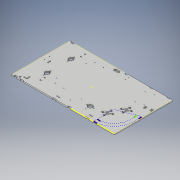
# Autodesk Inventor part: playfield
Saved by Autodesk Inventor 2017 (Build 210142000, 142)
## iProperties
Created: 2017-02-19
Part Number: playfield
Material: Generic
Document SubType Name: Modeling
Designer: John
Density: 1 g/cm^3
Appearance: Default
Author: John
Autodesk Inventor part; units mm, degrees
ref_plane "YZ Plane" through (0, 0, 0) normal (1, 0, 0) x (0, 1, 0)
ref_plane "XZ Plane" through (0, 0, 0) normal (0, 1, 0) x (-1, 0, 0)
ref_plane "XY Plane" through (0, 0, 0) normal (0, 0, 1) x (1, 0, 0)
sketch "Sketch2" plane through (0, 0, 0) normal (0, 1, 0) x (-1, 0, 0)
  line L0 (250, -141.5) -> (-250, -141.5)
  line L1 (-250, -141.5) -> (-250, 141.5)
  line L2 (-250, 141.5) -> (250, 141.5)
  line L3 (250, 141.5) -> (250, -141.5)
  line L4 (250, -141.5) -> (-250, 141.5) construction
  line L5 (-250, -141.5) -> (250, 141.5) construction
  line L6 (250, 138.5) -> (-250, 138.5) construction
  line L7 (250, 131.5) -> (-250, 131.5) construction
  line L8 (-250, 128.5) -> (250, 128.5) construction
  point P0 (0, 0)
  dimension "d0" = 500
  dimension "d1" = 283
  dimension "d4" = 3
  dimension "d5" = 7
  dimension "d6" = 3
  constraints: 18 end point, 6 point on line, 3 perpendicular, 2 horizontal, 2 midpoint, 2 parallel
  measures "d0" distance of L1.end L2.end
  measures "d1" distance of L0.end L1.end
  measures "d4" distance between parallel lines of L2 L6
  measures "d5" distance between parallel lines of L6 L7
  measures "d6" distance between parallel lines of L7 L8
extrude "Extrusion1" add sketch "Sketch2" along normal blind 6
sketch "Sketch3" plane through (0, 6, 0) normal (0, 1, 0) x (1, 0, 0)
  line L0 (-250, 141.5) -> (-250, -141.5) projected
  line L1 (-170, 66.5) -> (-170, -49.5) construction
  line L2 (-170, 66.5) -> (-170, 141.5) construction
  line L3 (250, 141.5) -> (-250, 141.5) construction
  line L4 (-170, -49.5) -> (-170, -141.5) construction
  line L5 (-250, -141.5) -> (250, -141.5) construction
  circle A0 centre (-170, 66.5) radius 10.825
  arc A1 (-169, 84.325) -> (-171, 84.325) centre (-170, 84.325) ccw
  line L6 (-170, 77.325) -> (-170, 84.325) construction
  line L7 (-169, 77.325) -> (-169, 84.325)
  line L8 (-171, 84.325) -> (-171, 77.325)
  arc A2 (-171, 77.325) -> (-169, 77.325) centre (-170, 77.325) ccw
  arc A3 (-169, 55.675) -> (-171, 55.675) centre (-170, 55.675) ccw
  line L9 (-169, 48.675) -> (-169, 55.675)
  arc A4 (-171, 48.675) -> (-169, 48.675) centre (-170, 48.675) ccw
  line L10 (-170, 55.675) -> (-170, 48.675) construction
  line L11 (-171, 55.675) -> (-171, 48.675)
  arc A5 (-169, -60.325) -> (-171, -60.325) centre (-170, -60.325) ccw
  arc A6 (-171, -38.675) -> (-169, -38.675) centre (-170, -38.675) ccw
  line L12 (-171, -31.675) -> (-171, -38.675)
  line L13 (-170, -38.675) -> (-170, -31.675) construction
  line L14 (-169, -38.675) -> (-169, -31.675)
  arc A7 (-169, -31.675) -> (-171, -31.675) centre (-170, -31.675) ccw
  circle A8 centre (-170, -49.5) radius 10.825
  arc A9 (-171, -67.325) -> (-169, -67.325) centre (-170, -67.325) ccw
  line L15 (-171, -60.325) -> (-171, -67.325)
  line L16 (-170, -60.325) -> (-170, -67.325) construction
  line L17 (-169, -67.325) -> (-169, -60.325)
  point P0 (0, 0)
  point P1 (-170, 80.825)
  point P2 (-170, 52.175)
  point P3 (-170, -35.175)
  point P4 (-170, -63.825)
  dimension "d8" = 49.5
  dimension "d12" = 116
  dimension "d134" = 80
  dimension "d173" = 21.65
  dimension "d174" = 7
  dimension "d175" = 2
  dimension "d176" = 7
  dimension "d177" = 2
  dimension "d178" = 21.65
  dimension "d179" = 7
  dimension "d180" = 2
  dimension "d181" = 7
  dimension "d182" = 2
  constraints: 38 end point, 20 point on circle, 16 tangent, 10 centre point, 6 vertical, 4 midpoint, 4 parallel, 2 point on line, 1 collinear
  measures "d8" vertical distance of point (0, 0) L1.end
  measures "d12" distance of L1.end L1.start
  measures "d134" distance from line of L1.start L0
  measures "d173" diameter of A0
  measures "d174" distance of L6.start L6.end
  measures "d175" diameter of A1
  measures "d176" distance of L10.start L10.end
  measures "d177" diameter of A4
  measures "d178" diameter of A8
  measures "d179" distance of L13.start L13.end
  measures "d180" diameter of A7
  measures "d181" distance of L16.start L16.end
  measures "d182" diameter of A9
extrude "Extrusion2" cut sketch "Sketch3" against normal through all
sketch "Sketch4" plane through (0, 6, 0) normal (0, 1, 0) x (1, 0, 0)
  circle A0 centre (-115, 85) radius 1.25
  circle A1 centre (-55, 110) radius 1.25
  circle A2 centre (-97, 110) radius 1.25
  line L0 (-250, 141.5) -> (-250, -141.5) construction
  circle A3 centre (-170, -49.5) radius 3.825 construction
  line L1 (-170, -49.5) -> (-170, 66.5) construction
  line L2 (-170, 8.5) -> (-250, 8.5) construction
  line L3 (-55, 110) -> (-115, 85) construction
  line L4 (-115, 85) -> (-97, 110) construction
  line L5 (-97, 110) -> (-55, 110) construction
  circle A4 centre (-107, -73) radius 1.25
  circle A5 centre (-65, -73) radius 1.25
  circle A6 centre (-125, -48) radius 1.25
  line L6 (-125, -48) -> (-107, -73) construction
  line L7 (-65, -73) -> (-125, -48) construction
  line L8 (-107, -73) -> (-65, -73) construction
  point P0 (0, 0)
  dimension "d16" = 2.5
  dimension "d24" = 2.5
  dimension "d34" = 2.5
  dimension "d39" = 60
  dimension "d41" = 25
  dimension "d55" = 110
  dimension "d60" = 25
  dimension "d61" = 55
  dimension "d62" = 18
  dimension "d284" = 45
  dimension "d285" = 1.5
  constraints: 16 end point, 6 centre point, 3 coincident, 1 midpoint, 1 perpendicular, 1 point on line, 1 vertical
  measures "d16" diameter of A0
  measures "d24" diameter of A1
  measures "d34" diameter of A2
  measures "d39" horizontal distance of L3.end L3.start
  measures "d41" vertical distance of L3.end L3.start
  measures "d55" vertical distance of point (0, 0) L3.start
  measures "d60" vertical distance of L3.end L4.end
  measures "d61" horizontal distance of L1.end L3.end
  measures "d62" horizontal distance of L3.end L4.end
  measures "d284" horizontal distance of L1.start A6.centre
  measures "d285" vertical distance of L1.start L6.start
extrude "Extrusion4" cut sketch "Sketch4" against normal through all
sketch "Sketch7" plane through (0, 6, 0) normal (0, 1, 0) x (1, 0, 0)
  line L0 (-250, 141.5) -> (-239.6, 141.5) construction
  line L1 (-239.6, 141.5) -> (-227.6, 141.5)
  line L2 (-227.6, 141.5) -> (-227.6, 135.5)
  line L3 (-227.6, 135.5) -> (-239.6, 135.5)
  line L4 (-239.6, 135.5) -> (-239.6, 141.5)
  line L5 (250, 141.5) -> (284.4, 141.5) construction
  line L6 (284.4, 141.5) -> (272.4, 141.5)
  line L7 (272.4, 141.5) -> (272.4, 138.5)
  line L8 (272.4, 138.5) -> (284.4, 138.5)
  line L9 (284.4, 138.5) -> (284.4, 141.5)
  line L10 (250, 141.5) -> (-250, 141.5) projected
  line L11 (34.4, 141.5) -> (22.4, 141.5)
  line L12 (22.4, 141.5) -> (22.4, 135.5)
  line L13 (22.4, 135.5) -> (34.4, 135.5)
  line L14 (34.4, 135.5) -> (34.4, 141.5)
  line L15 (250, -141.5) -> (-250, -141.5) projected
  line L16 (-239.6, -141.5) -> (-227.6, -141.5)
  line L17 (-227.6, -141.5) -> (-227.6, -135.5)
  line L18 (-227.6, -135.5) -> (-239.6, -135.5)
  line L19 (-239.6, -135.5) -> (-239.6, -141.5)
  line L20 (-250, 141.5) -> (-250, -141.5) projected
  line L21 (22.4, -141.5) -> (34.4, -141.5)
  line L22 (34.4, -141.5) -> (34.4, -135.5)
  line L23 (34.4, -135.5) -> (22.4, -135.5)
  line L24 (22.4, -135.5) -> (22.4, -141.5)
  line L25 (284.4, -141.5) -> (272.4, -141.5)
  line L26 (272.4, -141.5) -> (272.4, -135.5)
  line L27 (272.4, -135.5) -> (284.4, -135.5)
  line L28 (284.4, -135.5) -> (284.4, -141.5)
  line L29 (-250, -124.5) -> (-161, -124.5) construction
  line L30 (-161, -124.5) -> (-161, -141.5) construction
  line L31 (-250, -141.5) -> (250, -141.5) construction
  point P0 (0, 0)
  dimension "d104" = 10.4
  dimension "d105" = 12
  dimension "d106" = 6
  dimension "d108" = 12
  dimension "d109" = 3
  dimension "d112" = 500
  dimension "d113" = 12
  dimension "d114" = 6
  dimension "d115" = 250
  dimension "d116" = 12
  dimension "d117" = 6
  dimension "d118" = 10.4
  dimension "d123" = 12
  dimension "d124" = 12
  dimension "d125" = 500
  dimension "d126" = 250
  dimension "d127" = 17
  dimension "d128" = 89
  dimension "d283" = 6
  constraints: 56 end point, 13 parallel, 7 horizontal, 7 perpendicular, 6 point on line
  measures "d104" distance of L0.start L0.end
  measures "d105" distance of L2.end L3.end
  measures "d106" distance of L1.end L2.end
  measures "d108" distance of L8.end L7.end
  measures "d109" distance of L7.end L6.end
  measures "d112" distance between parallel lines of L7 L2
  measures "d113" distance of L13.end L12.end
  measures "d114" distance of L12.end L11.end
  measures "d115" distance between parallel lines of L2 L12
  measures "d116" distance of L18.end L17.end
  measures "d117" distance of L17.end L16.end
  measures "d118" distance between parallel lines of L20 L19
  measures "d123" distance of L23.end L22.end
  measures "d124" distance of L26.end L27.end
  measures "d125" distance between parallel lines of L17 L26
  measures "d126" distance between parallel lines of L24 L17
  measures "d127" distance of L29.end L30.end
  measures "d128" distance of L29.start L29.end
  measures "d283" distance of L23.end L21.start
extrude "Extrusion6" cut sketch "Sketch7" along normal through all both and the other way through all
sketch "Sketch8" plane through (0, 6, 0) normal (0, 1, 0) x (1, 0, 0)
  line L0 (147.3, -141.5) -> (147.3, -124.5) construction
  arc A0 (147.3, -124.5) -> (224.0343, -10.7368) centre (147.3, -41.7394) ccw construction
  line L1 (147.3, -41.7394) -> (147.3, -124.5) construction
  line L2 (147.3, -41.7394) -> (224.0343, -10.7368) construction
  line L3 (250, -141.5) -> (250, 141.5) construction
  arc A1 (147.3, -141.5) -> (239.7964, -4.3685) centre (147.3, -41.7394) ccw construction
  line L4 (147.3, -41.7394) -> (147.3, -141.5) construction
  line L5 (147.3, -41.7394) -> (239.7964, -4.3685) construction
  line L6 (22.4, 141.5) -> (-227.6, 141.5) construction
  line L7 (-250, 141.5) -> (-250, -141.5) construction
  line L8 (147.3, -124.5) -> (162.3, -124.5)
  line L9 (162.3, -124.5) -> (162.3, -121.5)
  line L10 (162.3, -121.5) -> (147.3, -121.5)
  line L11 (147.3, -121.5) -> (147.3, -124.5)
  line L12 (226.4695, -9.513) -> (223.688, -10.6368)
  line L13 (223.688, -10.6368) -> (229.3071, -24.5446)
  line L14 (229.3071, -24.5446) -> (232.0886, -23.4207)
  line L15 (232.0886, -23.4207) -> (226.4695, -9.513)
  line L16 (245.8953, -4.7279) -> (242.9409, -5.2488)
  line L17 (242.9409, -5.2488) -> (245.5456, -20.0209)
  line L18 (245.5456, -20.0209) -> (248.5, -19.5)
  line L19 (248.5, -19.5) -> (245.8953, -4.7279)
  line L20 (34.4, -141.5) -> (250, -141.5) projected
  line L21 (147.3, -141.5) -> (163.652, -141.5)
  line L22 (163.652, -141.5) -> (163.652, -138.5)
  line L23 (163.652, -138.5) -> (147.3, -138.5)
  line L24 (147.3, -138.5) -> (147.3, -141.5)
  point P0 (0, 0)
  dimension "d136" = 17
  dimension "d139" = 82.7606
  dimension "d142" = 112
  dimension "d146" = 112
  dimension "d183" = 15
  dimension "d184" = 3
  dimension "d185" = 3
  dimension "d186" = 15
  dimension "d189" = 22
  dimension "d190" = 3
  dimension "d191" = 15
  dimension "d193" = 100
  dimension "d194" = 1.5
  dimension "d195" = 122
  dimension "d196" = 3
  dimension "d197" = 17
  dimension "d198" = 397.3
  constraints: 42 end point, 8 parallel, 4 perpendicular, 4 point on circle, 2 centre point, 2 horizontal, 2 point on line, 2 vertical
  measures "d136" distance of L0.start L0.end
  measures "d139" radius of A0
  measures "d142" angle of L1 L2
  measures "d146" angle of L1 L5
  measures "d183" distance of L10.end L9.end
  measures "d184" distance of L9.end L8.end
  measures "d185" distance of L14.end L13.end
  measures "d186" distance of L13.end L12.end
  measures "d189" angle of L15 L3
  measures "d190" distance of L18.end L17.end
  measures "d191" distance of L17.end L16.end
  measures "d193" angle of L18 L3
  measures "d194" distance from line of L3 L18.end
  measures "d195" distance from line of L18.end L20
  measures "d196" distance of L22.end L21.end
  measures "d197" distance between parallel lines of L20 L8
  measures "d198" distance between parallel lines of L7 L24
extrude "Extrusion7" cut sketch "Sketch8" against normal blind 10
sketch "Sketch6" plane through (0, 6, 0) normal (0, 1, 0) x (1, 0, 0)
  line L0 (155.8231, -21.3423) -> (187, -39.3423) construction
  line L1 (187, -39.3423) -> (205, -8.1654) construction
  line L2 (205, -8.1654) -> (173.8231, 9.8346) construction
  line L3 (173.8231, 9.8346) -> (155.8231, -21.3423) construction
  line L4 (140.8231, -47.3231) -> (122.8231, -78.5) construction
  line L5 (122.8231, -78.5) -> (154, -96.5) construction
  line L6 (154, -96.5) -> (172, -65.3231) construction
  line L7 (172, -65.3231) -> (140.8231, -47.3231) construction
  line L8 (155.8231, -21.3423) -> (140.8231, -47.3231) construction
  line L9 (148.3231, -34.3327) -> (148.3231, -9.3327) construction
  line L10 (148.3231, -34.3327) -> (126.6725, -46.8327) construction
  line L11 (155.8231, -21.3423) -> (148.3231, -34.3327) construction
  line L12 (140.8231, -47.3231) -> (148.3231, -34.3327) construction
  line L13 (148.3231, -9.3327) -> (142.3231, -9.3327) construction
  line L14 (142.3231, -9.3327) -> (142.3231, -30.8686) construction
  line L15 (142.3231, -30.8686) -> (123.6725, -41.6366) construction
  line L16 (123.6725, -41.6366) -> (126.6725, -46.8327) construction
  line L17 (-250, -141.5) -> (250, -141.5) projected
  line L18 (250, 141.5) -> (250, -141.5) projected
  line L19 (21.5056, 88.4602) -> (-14.4944, 88.4602) construction
  line L20 (-14.4944, 88.4602) -> (-14.4944, 124.4602) construction
  line L21 (-14.4944, 124.4602) -> (21.5056, 124.4602) construction
  line L22 (21.5056, 124.4602) -> (21.5056, 88.4602) construction
  point P0 (0, 0)
  dimension "d78" = 36
  dimension "d79" = 36
  dimension "d80" = 36
  dimension "d81" = 36
  dimension "d82" = 30
  dimension "d83" = 25
  dimension "d87" = 6
  dimension "d89" = 45
  dimension "d98" = 45
  dimension "d99" = 30
  dimension "d101" = 30
  dimension "d147" = 36
  dimension "d148" = 36
  constraints: 42 end point, 6 parallel, 6 perpendicular, 3 equal length, 2 horizontal, 1 collinear, 1 midpoint, 1 vertical
  measures "d78" distance of L2.end L1.end
  measures "d79" distance of L1.end L0.end
  measures "d80" distance of L6.end L5.end
  measures "d81" distance of L5.end L4.end
  measures "d82" distance between parallel lines of L7 L0
  measures "d83" distance of L9.start L9.end
  measures "d87" distance of L9.end L13.end
  measures "d89" distance from line of L17 L5.end
  measures "d98" distance from line of L18 L1.end
  measures "d99" angle of L18 L1
  measures "d101" angle of L4 L10
  measures "d147" distance of L20.end L21.end
  measures "d148" distance of L19.end L20.end
sketch "Sketch10" plane through (0, 6, 0) normal (0, 1, 0) x (1, 0, 0)
  line L0 (250, -141.5) -> (250, 141.5) projected
  line L1 (205, -6.4334) -> (172.9571, 12.0666) construction
  line L2 (172.9571, 12.0666) -> (154.4571, -19.9763) construction
  line L3 (154.4571, -19.9763) -> (186.5, -38.4763) construction
  line L4 (186.5, -38.4763) -> (205, -6.4334) construction
  line L5 (195.75, -22.4548) -> (163.7071, -3.9548) construction
  line L6 (188.9785, 2.8166) -> (170.4785, -29.2263) construction
  line L7 (186.5, -38.4763) -> (172.9571, 12.0666) construction
  line L8 (205, -6.4334) -> (154.4571, -19.9763) construction
  circle A0 centre (179.7285, -13.2048) radius 3.5
  line L9 (201.2859, -4.8664) -> (193.4917, -0.3664)
  line L10 (193.4917, -0.3664) -> (190.4917, -5.5625)
  line L11 (190.4917, -5.5625) -> (198.2859, -10.0625)
  line L12 (198.2859, -10.0625) -> (201.2859, -4.8664)
  line L13 (201.2859, -4.8664) -> (195.8888, -5.2144) construction
  line L14 (193.4917, -0.3664) -> (195.8888, -5.2144) construction
  line L15 (195.8888, -5.2144) -> (198.2859, -10.0625) construction
  line L16 (195.8888, -5.2144) -> (190.4917, -5.5625) construction
  circle A1 centre (187.9247, -11.0087) radius 2.5
  circle A2 centre (187.0897, -17.4548) radius 1.5
  line L17 (183.2859, -36.0433) -> (175.4917, -31.5433)
  line L18 (175.4917, -31.5433) -> (178.4917, -26.3471)
  line L19 (178.4917, -26.3471) -> (186.2859, -30.8471)
  line L20 (186.2859, -30.8471) -> (183.2859, -36.0433)
  line L21 (183.2859, -36.0433) -> (180.8888, -31.1952) construction
  line L22 (175.4917, -31.5433) -> (180.8888, -31.1952) construction
  line L23 (180.8888, -31.1952) -> (186.2859, -30.8471) construction
  line L24 (180.8888, -31.1952) -> (178.4917, -26.3471) construction
  circle A3 centre (181.9247, -21.401) radius 2.5
  circle A4 centre (187.0897, -17.4548) radius 1.5
  line L25 (176.1712, 9.6336) -> (183.9654, 5.1336)
  line L26 (183.9654, 5.1336) -> (180.9654, -0.0625)
  line L27 (180.9654, -0.0625) -> (173.1712, 4.4375)
  line L28 (173.1712, 4.4375) -> (176.1712, 9.6336)
  line L29 (176.1712, 9.6336) -> (178.5683, 4.7856) construction
  line L30 (183.9654, 5.1336) -> (178.5683, 4.7856) construction
  line L31 (178.5683, 4.7856) -> (173.1712, 4.4375) construction
  line L32 (178.5683, 4.7856) -> (180.9654, -0.0625) construction
  circle A5 centre (177.5324, -5.0087) radius 2.5
  circle A6 centre (172.3673, -8.9548) radius 1.5
  line L33 (158.1712, -21.5433) -> (165.9654, -26.0433)
  line L34 (165.9654, -26.0433) -> (163.5683, -21.1952) construction
  line L35 (158.1712, -21.5433) -> (163.5683, -21.1952) construction
  line L36 (163.5683, -21.1952) -> (168.9654, -20.8471) construction
  line L37 (165.9654, -26.0433) -> (168.9654, -20.8471)
  line L38 (168.9654, -20.8471) -> (161.1712, -16.3471)
  line L39 (161.1712, -16.3471) -> (158.1712, -21.5433)
  line L40 (163.5683, -21.1952) -> (161.1712, -16.3471) construction
  circle A7 centre (171.5324, -15.401) radius 2.5
  circle A8 centre (172.3673, -8.9548) radius 1.5
  line L41 (171.5, -64.4571) -> (139.4571, -45.9571) construction
  line L42 (139.4571, -45.9571) -> (120.9571, -78) construction
  line L43 (120.9571, -78) -> (153, -96.5) construction
  line L44 (153, -96.5) -> (171.5, -64.4571) construction
  line L45 (162.25, -80.4785) -> (130.2071, -61.9785) construction
  line L46 (155.4785, -55.2071) -> (136.9785, -87.25) construction
  line L47 (153, -96.5) -> (139.4571, -45.9571) construction
  line L48 (171.5, -64.4571) -> (120.9571, -78) construction
  circle A9 centre (146.2285, -71.2285) radius 3.5
  line L49 (167.7859, -62.8901) -> (159.9917, -58.3901)
  line L50 (159.9917, -58.3901) -> (156.9917, -63.5862)
  line L51 (156.9917, -63.5862) -> (164.7859, -68.0862)
  line L52 (164.7859, -68.0862) -> (167.7859, -62.8901)
  line L53 (167.7859, -62.8901) -> (162.3888, -63.2381) construction
  line L54 (159.9917, -58.3901) -> (162.3888, -63.2381) construction
  line L55 (162.3888, -63.2381) -> (164.7859, -68.0862) construction
  line L56 (162.3888, -63.2381) -> (156.9917, -63.5862) construction
  circle A10 centre (154.4247, -69.0324) radius 2.5
  circle A11 centre (153.5897, -75.4785) radius 1.5
  line L57 (149.7859, -94.067) -> (141.9917, -89.567)
  line L58 (141.9917, -89.567) -> (147.3888, -89.2189) construction
  line L59 (149.7859, -94.067) -> (147.3888, -89.2189) construction
  line L60 (147.3888, -89.2189) -> (144.9917, -84.3708) construction
  line L61 (141.9917, -89.567) -> (144.9917, -84.3708)
  line L62 (144.9917, -84.3708) -> (152.7859, -88.8708)
  line L63 (152.7859, -88.8708) -> (149.7859, -94.067)
  line L64 (147.3888, -89.2189) -> (152.7859, -88.8708) construction
  circle A12 centre (148.4247, -79.4247) radius 2.5
  circle A13 centre (153.5897, -75.4785) radius 1.5
  circle A14 centre (138.8673, -66.9785) radius 1.5
  circle A15 centre (138.8673, -66.9785) radius 1.5
  circle A16 centre (144.0324, -63.0324) radius 2.5
  line L65 (145.0683, -53.2381) -> (147.4654, -58.0862) construction
  line L66 (147.4654, -58.0862) -> (139.6712, -53.5862)
  line L67 (145.0683, -53.2381) -> (139.6712, -53.5862) construction
  line L68 (150.4654, -52.8901) -> (147.4654, -58.0862)
  line L69 (139.6712, -53.5862) -> (142.6712, -48.3901)
  line L70 (142.6712, -48.3901) -> (145.0683, -53.2381) construction
  line L71 (150.4654, -52.8901) -> (145.0683, -53.2381) construction
  line L72 (142.6712, -48.3901) -> (150.4654, -52.8901)
  circle A17 centre (138.0324, -73.4247) radius 2.5
  line L73 (127.6712, -74.3708) -> (124.6712, -79.567)
  line L74 (130.0683, -79.2189) -> (127.6712, -74.3708) construction
  line L75 (124.6712, -79.567) -> (130.0683, -79.2189) construction
  line L76 (135.4654, -78.8708) -> (127.6712, -74.3708)
  line L77 (130.0683, -79.2189) -> (135.4654, -78.8708) construction
  line L78 (124.6712, -79.567) -> (132.4654, -84.067)
  line L79 (132.4654, -84.067) -> (130.0683, -79.2189) construction
  line L80 (132.4654, -84.067) -> (135.4654, -78.8708)
  line L81 (34.4, -141.5) -> (250, -141.5) projected
  dimension "d253" = 37
  dimension "d254" = 37
  dimension "d255" = 7
  dimension "d256" = 9
  dimension "d257" = 6
  dimension "d258" = 14.5
  dimension "d261" = 12
  dimension "d262" = 5
  dimension "d263" = 6
  dimension "d264" = 3
  dimension "d265" = 8.5
  dimension "d266" = 45
  dimension "d267" = 30
  dimension "d268" = 37
  dimension "d269" = 37
  dimension "d270" = 7
  dimension "d271" = 9
  dimension "d272" = 6
  dimension "d273" = 14.5
  dimension "d274" = 12
  dimension "d275" = 5
  dimension "d276" = 6
  dimension "d277" = 3
  dimension "d278" = 8.5
  dimension "d279" = 30
  dimension "d280" = 45
  constraints: 160 end point, 38 symmetric about line, 18 centre point, 10 midpoint, 8 parallel, 5 collinear, 4 perpendicular, 4 point on line, 12 other
  measures "d253" distance of L3.end L2.end
  measures "d254" distance of L2.end L1.end
  measures "d255" diameter of A0
  measures "d256" distance of L11.end L10.end
  measures "d257" distance of L10.end L9.end
  measures "d258" distance between parallel lines of L12 L6
  measures "d261" distance between parallel lines of L11 L5
  measures "d262" diameter of A1
  measures "d263" distance from line of A1.centre L6
  measures "d264" diameter of A2
  measures "d265" distance from line of L6 A2.centre
  measures "d266" distance from line of L0 L1.start
  measures "d267" angle of L4 L0
  measures "d268" distance of L47.start L42.end
  measures "d269" distance of L42.end L47.end
  measures "d270" diameter of A9
  measures "d271" distance of L51.end L50.end
  measures "d272" distance of L50.end L50.start
  measures "d273" distance between parallel lines of L52 L46
  measures "d274" distance between parallel lines of L51 L45
  measures "d275" diameter of A10
  measures "d276" distance from line of A10.centre L46
  measures "d277" diameter of A11
  measures "d278" distance from line of L46 A11.centre
  measures "d279" distance between parallel lines of L3 L41
  measures "d280" distance from line of L81 L47.start
extrude "Extrusion8" cut sketch "Sketch10" against normal through all
sketch "servo" plane through (0, 6, 0) normal (0, 1, 0) x (1, 0, 0)
  line L0 (2, 134.5) -> (-19.846, 134.5)
  line L1 (-19.846, 134.5) -> (-19.846, 123.375)
  line L2 (-19.846, 123.375) -> (2, 123.375)
  line L3 (2, 123.375) -> (2, 134.5)
  line L4 (-250, 141.5) -> (-250, -141.5) projected
  line L5 (-227.6, 141.5) -> (22.4, 141.5) projected
  line L6 (-19.846, 134.5) -> (-23.923, 134.5)
  line L7 (-23.923, 134.5) -> (-23.923, 123.375)
  line L8 (-23.923, 123.375) -> (-19.846, 123.375)
  line L9 (-19.846, 123.375) -> (-19.846, 134.5)
  line L10 (2, 134.5) -> (6.077, 134.5)
  line L11 (6.077, 134.5) -> (6.077, 123.375)
  line L12 (6.077, 123.375) -> (2, 123.375)
  line L13 (2, 123.375) -> (2, 134.5)
  circle A0 centre (-21.8845, 128.9375) radius 1
  circle A1 centre (4.0385, 128.9375) radius 1
  line L14 (6.077, 134.5) -> (4.0385, 128.9375) construction
  line L15 (2, 134.5) -> (4.0385, 128.9375) construction
  line L16 (4.0385, 128.9375) -> (2, 123.375) construction
  line L17 (4.0385, 128.9375) -> (6.077, 123.375) construction
  line L18 (-19.846, 134.5) -> (-23.923, 123.375) construction
  line L19 (-23.923, 134.5) -> (-19.846, 123.375) construction
  point P0 (0, 0)
  dimension "d286" = 252
  dimension "d288" = 11.125
  dimension "d289" = 7
  dimension "d290" = 4.077
  dimension "d291" = 4.077
  dimension "d292" = 2
  dimension "d293" = 2
  dimension "d296" = 30
  constraints: 36 end point, 6 parallel, 3 collinear, 3 horizontal, 3 perpendicular, 2 centre point, 2 coincident, 1 midpoint, 1 point on line
  measures "d286" distance between parallel lines of L4 L3
  measures "d288" distance between parallel lines of L2 L0
  measures "d289" distance between parallel lines of L5 L0
  measures "d290" distance of L8.end L7.end
  measures "d291" distance of L11.end L12.end
  measures "d292" diameter of A0
  measures "d293" diameter of A1
  measures "d296" distance between parallel lines of L7 L11
extrude "Extrusion9" cut sketch "servo" against normal blind 10 contours L3 L2 L1 L0 | A0 | A1
sketch "Sketch12" plane through (0, 6, 0) normal (0, 1, 0) x (1, 0, 0)
  line L0 (-222.6, -134.5) -> (-216.6, -134.5)
  line L1 (-216.6, -134.5) -> (-216.6, -128.5)
  line L2 (-216.6, -128.5) -> (-222.6, -128.5)
  line L3 (-222.6, -128.5) -> (-222.6, -134.5)
  line L4 (-227.6, -141.5) -> (22.4, -141.5) projected
  line L5 (-250, 141.5) -> (-250, -141.5) projected
  line L6 (-227.6, -135.5) -> (-227.6, -141.5) projected
  point P0 (0, 0)
  dimension "d297" = 6
  dimension "d298" = 6
  dimension "d299" = 7
  dimension "d301" = 5
  constraints: 8 end point, 2 parallel, 1 horizontal, 1 perpendicular
  measures "d297" distance of L2.end L1.end
  measures "d298" distance of L1.end L0.end
  measures "d299" distance between parallel lines of L4 L0
  measures "d301" distance between parallel lines of L3 L6
extrude "Extrusion10" cut sketch "Sketch12" along normal through all both and the other way through all
sketch "Sketch13" plane through (0, 6, 0) normal (0, 1, 0) x (1, 0, 0)
  circle A0 centre (0, -107) radius 1.25
  circle A1 centre (23.5, -76.5) radius 1.25
  circle A2 centre (75.5, -107) radius 1.25
  line L0 (-227.6, -141.5) -> (22.4, -141.5) projected
  line L1 (34.4, -141.5) -> (147.3, -141.5) projected
  line L2 (-250, 141.5) -> (-250, -141.5) projected
  arc A3 (87.0662, -83.9826) -> (87.0662, -85.9826) centre (87.0662, -84.9826) ccw
  arc A4 (65.4162, -85.9826) -> (65.4162, -83.9826) centre (65.4162, -84.9826) ccw
  line L3 (58.4162, -85.9826) -> (65.4162, -85.9826)
  line L4 (65.4162, -84.9826) -> (58.4162, -84.9826) construction
  line L5 (65.4162, -83.9826) -> (58.4162, -83.9826)
  arc A5 (58.4162, -83.9826) -> (58.4162, -85.9826) centre (58.4162, -84.9826) ccw
  circle A6 centre (76.2412, -84.9826) radius 10.825
  arc A7 (94.0662, -85.9826) -> (94.0662, -83.9826) centre (94.0662, -84.9826) ccw
  line L6 (87.0662, -85.9826) -> (94.0662, -85.9826)
  line L7 (87.0662, -84.9826) -> (94.0662, -84.9826) construction
  line L8 (94.0662, -83.9826) -> (87.0662, -83.9826)
  point P0 (0, 0)
  point P1 (76.2412, -84.9826)
  point P2 (61.9162, -84.9826)
  point P3 (90.5662, -84.9826)
  dimension "d304" = 2.5
  dimension "d305" = 2.5
  dimension "d306" = 2.5
  dimension "d307" = 34.5
  dimension "d308" = 34.5
  dimension "d309" = 30.5
  dimension "d310" = 75.5
  dimension "d311" = 23.5
  dimension "d312" = 250
  dimension "d377" = 21.65
  dimension "d378" = 7
  dimension "d379" = 2
  dimension "d380" = 7
  dimension "d381" = 2
  constraints: 16 end point, 10 point on circle, 8 centre point, 8 tangent, 2 midpoint, 2 parallel
  measures "d304" diameter of A0
  measures "d305" diameter of A1
  measures "d306" diameter of A2
  measures "d307" distance from line of L0 A0.centre
  measures "d308" distance from line of L1 A2.centre
  measures "d309" vertical distance of A0.centre A1.centre
  measures "d310" distance of A2.centre A0.centre
  measures "d311" horizontal distance of A0.centre A1.centre
  measures "d312" distance from line of L2 A0.centre
  measures "d377" diameter of A6
  measures "d378" distance of L4.start L4.end
  measures "d379" diameter of A5
  measures "d380" distance of L7.start L7.end
  measures "d381" diameter of A7
extrude "Extrusion11" cut sketch "Sketch13" against normal through all
sketch "Sketch14" plane through (0, 6, 0) normal (0, 1, 0) x (1, 0, 0)
  circle A0 centre (-234.5, 26.5) radius 1.25
  circle A1 centre (-234.5, 1.5) radius 1.25
  line L0 (-250, 141.5) -> (-250, -141.5) projected
  line L1 (-239.6, 141.5) -> (-250, 141.5) projected
  point P0 (0, 0)
  dimension "d315" = 2.5
  dimension "d316" = 2.5
  dimension "d317" = 25
  dimension "d318" = 15.5
  dimension "d319" = 115
  dimension "d320" = 15.5
  constraints: 2 centre point
  measures "d315" diameter of A0
  measures "d316" diameter of A1
  measures "d317" distance of A1.centre A0.centre
  measures "d318" distance from line of L0 A0.centre
  measures "d319" distance from line of A0.centre L1
  measures "d320" distance from line of L0 A1.centre
sketch "Sketch15" plane through (0, 6, 0) normal (0, 1, 0) x (1, 0, 0)
  circle A0 centre (183.5, 119) radius 1.25
  circle A1 centre (201.3585, 52.3511) radius 1.25
  circle A2 centre (148.7267, 109.6825) radius 1.25
  circle A3 centre (166.5852, 43.0336) radius 1.25
  line L0 (183.5, 119) -> (201.3585, 52.3511) construction
  line L1 (201.3585, 52.3511) -> (166.5852, 43.0336) construction
  line L2 (166.5852, 43.0336) -> (148.7267, 109.6825) construction
  line L3 (148.7267, 109.6825) -> (183.5, 119) construction
  line L4 (250, 141.5) -> (34.4, 141.5) construction
  line L5 (250, -141.5) -> (250, 141.5) construction
  line L6 (247.085, 43.1) -> (238.2217, 41.5372)
  line L7 (238.2217, 41.5372) -> (236.138, 53.3549)
  line L8 (236.138, 53.3549) -> (245.0012, 54.9177)
  line L9 (245.0012, 54.9177) -> (247.085, 43.1)
  line L10 (218.4114, 50.2292) -> (209.5481, 48.6664)
  line L11 (209.5481, 48.6664) -> (211.6319, 36.8487)
  line L12 (211.6319, 36.8487) -> (220.4952, 38.4115)
  line L13 (220.4952, 38.4115) -> (218.4114, 50.2292)
  circle A4 centre (47.9, 128.5) radius 1.25
  circle A5 centre (47.9, 113.5) radius 1.25
  line L14 (34.4, 141.5) -> (34.4, 135.5) projected
  point P0 (0, 0)
  dimension "d321" = 2.5
  dimension "d322" = 2.5
  dimension "d323" = 2.5
  dimension "d324" = 2.5
  dimension "d325" = 36
  dimension "d326" = 36
  dimension "d327" = 69
  dimension "d328" = 22.5
  dimension "d329" = 66.5
  dimension "d330" = 105
  dimension "d331" = 9
  dimension "d332" = 12
  dimension "d333" = 80
  dimension "d334" = 2.915
  dimension "d335" = 98.4
  dimension "d336" = 9
  dimension "d337" = 12
  dimension "d338" = 18
  dimension "d343" = 2.5
  dimension "d344" = 2.5
  dimension "d345" = 15
  dimension "d346" = 13
  dimension "d347" = 13.5
  dimension "d348" = 13.5
  constraints: 24 end point, 6 centre point, 5 parallel, 4 perpendicular, 1 collinear
  measures "d321" diameter of A0
  measures "d322" diameter of A1
  measures "d323" diameter of A2
  measures "d324" diameter of A3
  measures "d325" distance of L2.end L0.start
  measures "d326" distance of L1.end L0.end
  measures "d327" distance of L0.end L0.start
  measures "d328" distance from line of L4 L0.start
  measures "d329" distance from line of L5 L0.start
  measures "d330" angle of L0 L4
  measures "d331" distance of L7.end L8.end
  measures "d332" distance of L6.end L7.end
  measures "d333" angle of L5 L6
  measures "d334" distance from line of L5 L6.start
  measures "d335" distance from line of L4 L6.start
  measures "d336" distance of L12.end L11.end
  measures "d337" distance of L11.end L10.end
  measures "d338" distance between parallel lines of L13 L7
  measures "d343" diameter of A4
  measures "d344" diameter of A5
  measures "d345" distance of A5.centre A4.centre
  measures "d346" distance from line of L4 A4.centre
  measures "d347" distance from line of L14 A4.centre
  measures "d348" distance from line of L14 A5.centre
extrude "Extrusion12" cut sketch "Sketch15" along normal through all both and the other way through all
extrude "Extrusion13" cut sketch "Sketch14" along normal through all both and the other way through all
sketch "Sketch16" plane through (0, 6, 0) normal (0, 1, 0) x (1, 0, 0)
  circle A0 centre (-156.2, 121.5) radius 1.25
  circle A1 centre (-156.2, 101.5) radius 1.25
  line L0 (22.4, 141.5) -> (-227.6, 141.5) projected
  line L1 (-250, 141.5) -> (-250, -141.5) projected
  line L2 (-156.2, 121.5) -> (-156.2, 101.5) construction
  circle A2 centre (-156.2, -75.416) radius 1.25
  circle A3 centre (-156.2, -95.416) radius 1.25
  line L3 (-156.2, -75.416) -> (-156.2, -95.416) construction
  line L4 (-227.6, -141.5) -> (22.4, -141.5) construction
  line L5 (-153.5089, 121.5) -> (-158.5089, 121.5) construction
  line L6 (-153.5089, 122.75) -> (-158.5089, 122.75)
  line L7 (-158.5089, 120.25) -> (-153.5089, 120.25)
  arc A4 (-153.5089, 120.25) -> (-153.5089, 122.75) centre (-153.5089, 121.5) ccw
  arc A5 (-158.5089, 122.75) -> (-158.5089, 120.25) centre (-158.5089, 121.5) ccw
  line L8 (-152.9621, 101.5) -> (-157.9621, 101.5) construction
  line L9 (-152.9621, 102.75) -> (-157.9621, 102.75)
  line L10 (-157.9621, 100.25) -> (-152.9621, 100.25)
  arc A6 (-152.9621, 100.25) -> (-152.9621, 102.75) centre (-152.9621, 101.5) ccw
  arc A7 (-157.9621, 102.75) -> (-157.9621, 100.25) centre (-157.9621, 101.5) ccw
  line L11 (-152.9621, 101.5) -> (-147.9621, 101.5) construction
  line L12 (-152.9621, -75.416) -> (-157.9621, -75.416) construction
  line L13 (-152.9621, -74.166) -> (-157.9621, -74.166)
  line L14 (-157.9621, -76.666) -> (-152.9621, -76.666)
  arc A8 (-152.9621, -76.666) -> (-152.9621, -74.166) centre (-152.9621, -75.416) ccw
  arc A9 (-157.9621, -74.166) -> (-157.9621, -76.666) centre (-157.9621, -75.416) ccw
  line L15 (-152.9621, 101.5) -> (-152.9621, -75.416) construction
  line L16 (-152.9621, -95.416) -> (-157.9621, -95.416) construction
  line L17 (-152.9621, -94.166) -> (-157.9621, -94.166)
  line L18 (-157.9621, -96.666) -> (-152.9621, -96.666)
  arc A10 (-152.9621, -96.666) -> (-152.9621, -94.166) centre (-152.9621, -95.416) ccw
  arc A11 (-157.9621, -94.166) -> (-157.9621, -96.666) centre (-157.9621, -95.416) ccw
  point P0 (0, 0)
  point P1 (-156.0089, 121.5)
  point P2 (-155.4621, 101.5)
  point P3 (-155.4621, -75.416)
  point P4 (-155.4621, -95.416)
  dimension "d349" = 2.5
  dimension "d350" = 2.5
  dimension "d351" = 20
  dimension "d352" = 20
  dimension "d353" = 93.8
  dimension "d356" = 2.5
  dimension "d357" = 2.5
  dimension "d358" = 20
  dimension "d359" = 46.084
  dimension "d360" = 5
  dimension "d361" = 2.5
  dimension "d362" = 5
  dimension "d363" = 180
  dimension "d364" = 2.5
  dimension "d365" = 20
  dimension "d368" = 5
  dimension "d369" = 2.5
  dimension "d370" = 5
  dimension "d371" = 2.5
  constraints: 40 end point, 17 tangent, 16 point on circle, 12 centre point, 4 horizontal, 4 midpoint, 4 parallel, 3 vertical, 2 collinear, 1 perpendicular
  measures "d349" diameter of A0
  measures "d350" diameter of A1
  measures "d351" distance of L2.end L2.start
  measures "d352" distance from line of L2.start L0
  measures "d353" distance from line of L1 L2.start
  measures "d356" diameter of A2
  measures "d357" diameter of A3
  measures "d358" distance of L3.start L3.end
  measures "d359" distance from line of L4 L3.end
  measures "d360" distance of L5.start L5.end
  measures "d361" diameter of A5
  measures "d362" distance of L8.start L8.end
  measures "d363" angle of L8 L11
  measures "d364" diameter of A7
  measures "d365" distance between parallel lines of L8 L5
  measures "d368" distance of L12.start L12.end
  measures "d369" diameter of A9
  measures "d370" distance of L16.start L16.end
  measures "d371" diameter of A11
extrude "Extrusion14" cut sketch "Sketch16" along normal through all both and the other way through all
sketch "Sketch17" plane through (0, 6, 0) normal (0, 1, 0) x (1, 0, 0)
  line L0 (250, 141.5) -> (34.4, 141.5) projected
  line L1 (238, 141.5) -> (226, 141.5)
  line L2 (226, 141.5) -> (226, 138.5)
  line L3 (226, 138.5) -> (238, 138.5)
  line L4 (238, 138.5) -> (238, 141.5)
  line L5 (154, 141.5) -> (142, 141.5)
  line L6 (142, 141.5) -> (142, 138.5)
  line L7 (142, 138.5) -> (154, 138.5)
  line L8 (154, 138.5) -> (154, 141.5)
  line L9 (250, -141.5) -> (250, 141.5) projected
  point P0 (0, 0)
  dimension "d382" = 12
  dimension "d383" = 3
  dimension "d384" = 12
  dimension "d385" = 3
  dimension "d386" = 72
  dimension "d387" = 12
  constraints: 16 end point, 4 parallel, 2 horizontal, 2 perpendicular, 2 point on line
  measures "d382" distance of L3.end L2.end
  measures "d383" distance of L2.end L1.end
  measures "d384" distance of L7.end L6.end
  measures "d385" distance of L6.end L5.end
  measures "d386" distance between parallel lines of L8 L2
  measures "d387" distance between parallel lines of L4 L9
extrude "Extrusion15" cut sketch "Sketch17" against normal through all
sketch "Sketch18" plane through (0, 6, 0) normal (0, 1, 0) x (1, 0, 0)
  line L0 (-227.6, -141.5) -> (22.4, -141.5) projected
  line L1 (-250, 141.5) -> (-250, -141.5) projected
  line L2 (-193.3852, -121.0825) -> (-195.4728, -106.2285)
  line L3 (-196.356, -121.5) -> (-198.4436, -106.646)
  line L4 (-195.4728, -106.2285) -> (-198.4436, -106.646)
  line L5 (-196.356, -121.5) -> (-193.3852, -121.0825)
  line L6 (-209.6684, -5.2211) -> (-211.756, 9.6329)
  line L7 (-211.756, 9.6329) -> (-214.7268, 9.2154)
  line L8 (-214.7268, 9.2154) -> (-212.6393, -5.6386)
  line L9 (-212.6393, -5.6386) -> (-209.6684, -5.2211)
  point P0 (0, 0)
  dimension "d394" = 15
  dimension "d395" = 98
  dimension "d396" = 15
  dimension "d397" = 3
  dimension "d398" = 20
  dimension "d399" = 53.644
  dimension "d402" = 15
  dimension "d403" = 3
  dimension "d404" = 102
  constraints: 16 end point, 4 perpendicular, 1 parallel
  measures "d394" distance of L2.start L2.end
  measures "d395" angle of L0 L2
  measures "d396" distance of L3.start L3.end
  measures "d397" distance of L2.end L3.end
  measures "d398" distance from line of L0 L3.start
  measures "d399" distance from line of L1 L3.start
  measures "d402" distance of L6.start L6.end
  measures "d403" distance of L6.end L7.end
  measures "d404" distance between parallel lines of L4 L9
extrude "Extrusion16" cut sketch "Sketch18" along normal through all both and the other way through all
sketch "Sketch19" plane through (0, 6, 0) normal (0, 1, 0) x (1, 0, 0)
  line L0 (-227.6, -141.5) -> (22.4, -141.5) projected
  line L1 (-210, -141.5) -> (-195, -141.5)
  line L2 (-195, -141.5) -> (-195, -138.5)
  line L3 (-195, -138.5) -> (-210, -138.5)
  line L4 (-210, -138.5) -> (-210, -141.5)
  line L5 (-250, 141.5) -> (-250, -141.5) projected
  line L6 (125, -141.5) -> (110, -141.5)
  line L7 (110, -141.5) -> (110, -138.5)
  line L8 (110, -138.5) -> (125, -138.5)
  line L9 (125, -138.5) -> (125, -141.5)
  line L10 (-35, -141.5) -> (-50, -141.5)
  line L11 (-50, -141.5) -> (-50, -138.5)
  line L12 (-50, -138.5) -> (-35, -138.5)
  line L13 (-35, -138.5) -> (-35, -141.5)
  line L14 (-195, -124.5) -> (-210, -124.5)
  line L15 (-210, -124.5) -> (-210, -121.5)
  line L16 (-210, -121.5) -> (-195, -121.5)
  line L17 (-195, -121.5) -> (-195, -124.5)
  line L18 (-35, -124.5) -> (-50, -124.5)
  line L19 (-50, -124.5) -> (-50, -121.5)
  line L20 (-50, -121.5) -> (-35, -121.5)
  line L21 (-35, -121.5) -> (-35, -124.5)
  line L22 (125, -124.5) -> (110, -124.5)
  line L23 (110, -124.5) -> (110, -121.5)
  line L24 (110, -121.5) -> (125, -121.5)
  line L25 (125, -121.5) -> (125, -124.5)
  point P0 (0, 0)
  dimension "d406" = 15
  dimension "d407" = 3
  dimension "d408" = 40
  dimension "d409" = 15
  dimension "d410" = 15
  dimension "d411" = 145
  dimension "d412" = 145
  dimension "d415" = 15
  dimension "d416" = 3
  dimension "d417" = 14
  dimension "d418" = 15
  dimension "d419" = 3
  dimension "d420" = 14
  dimension "d421" = 3
  dimension "d422" = 3
  dimension "d423" = 14
  dimension "d424" = 15
  constraints: 48 end point, 12 parallel, 6 horizontal, 6 perpendicular, 4 point on line, 3 collinear
  measures "d406" distance of L3.end L2.end
  measures "d407" distance of L2.end L1.end
  measures "d408" distance between parallel lines of L5 L4
  measures "d409" distance of L7.end L8.end
  measures "d410" distance of L11.end L12.end
  measures "d411" distance between parallel lines of L13 L7
  measures "d412" distance between parallel lines of L2 L11
  measures "d415" distance of L15.end L16.end
  measures "d416" distance of L14.end L15.end
  measures "d417" distance between parallel lines of L3 L14
  measures "d418" distance of L19.end L20.end
  measures "d419" distance of L18.end L19.end
  measures "d420" distance between parallel lines of L12 L18
  measures "d421" distance of L12.end L10.start
  measures "d422" distance of L22.end L23.end
  measures "d423" distance between parallel lines of L8 L22
  measures "d424" distance of L23.end L24.end
extrude "Extrusion17" cut sketch "Sketch19" against normal through all
equation "\"d79\" = d78"
equation "\"d80\" = d78"
equation "\"d81\" = d78"
body "Solid1"
